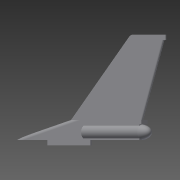
# Autodesk Inventor part: stabillizer
Saved by Autodesk Inventor 2014 SP1 (Build 180222100, 222)
## iProperties
Created: 2018-05-06
Part Number: stabillizer
Material: Generic
Document SubType Name: Modeling
Designer: Dadang
Density: 1 g/cm^3
Appearance: Default
Author: Dadang
Autodesk Inventor part; units mm, degrees
ref_plane "YZ Plane" through (0, 0, 0) normal (1, 0, 0) x (0, 1, 0)
ref_plane "XZ Plane" through (0, 0, 0) normal (0, 1, 0) x (-1, 0, 0)
sketch "Sketch1" plane through (0, 0, 0) normal (0, 0, 1) x (1, 0, 0)
  line L0 (0, 0) -> (330, 0)
  line L1 (0, 0) -> (0, 28)
  line L2 (0, 28) -> (-5, 28)
  line L3 (-5, 28) -> (-5, 36)
  line L4 (-5, 36) -> (183, 36)
  line L5 (183, 36) -> (330, 0)
  line L6 (-60, 191) -> (-60, 181)
  line L7 (-60, 181) -> (-55, 181)
  line L8 (-55, 181) -> (0, 36)
  line L9 (-60, 191) -> (25, 191)
  line L10 (33.5125, 187.4416) -> (183, 36)
  line L11 (25, 191) -> (33.5125, 187.4416)
  line L12 (242, 0) -> (242, -10)
  line L13 (242, -10) -> (132, -10)
  line L14 (132, -10) -> (132, 0)
  point P0 (30, 191)
  dimension "d0" = 330
  dimension "d1" = 28
  dimension "d2" = 5
  dimension "d3" = 8
  dimension "d4" = 188
  dimension "d7" = 10
  dimension "d8" = 5
  dimension "d9" = 90
  dimension "d10" = 88
  dimension "d11" = 10
  dimension "d12" = 110
  dimension "d23" = 145
  constraints: 30 end point, 5 point on line, 4 perpendicular, 3 parallel, 1 horizontal
  measures "d0" distance of L0.start L0.end
  measures "d1" distance of L0.start L1.end
  measures "d2" distance of L1.end L2.end
  measures "d3" distance of L2.end L3.end
  measures "d4" distance of L3.end L4.end
  measures "d7" distance of L6.start L6.end
  measures "d8" distance of L6.end L7.end
  measures "d9" distance of L6.start point (30, 191)
  measures "d10" distance of L0.end L12.start
  measures "d11" distance of L12.start L12.end
  measures "d12" distance of L12.end L13.end
  measures "d23" vertical distance of L7.end L8.end
extrude "Extrusion1" add sketch "Sketch1" along normal mid plane 16 contours L1 L2 L3 L4 L5 L0
extrude "Extrusion2" add sketch "Sketch1" along normal mid plane 5 contours L0 L12 L13 L14 | L4 L8 L7 L6 L9 L11 L10
fillet "Fillet1" radius 2.5 6 edges at (108.2563, 111.7208, 2.5) (108.2563, 111.7208, -2.5) (-60, 186, 2.5) (-60, 186, -2.5) (-27.5, 108.5, 2.5) (-27.5, 108.5, -2.5)
sketch "Sketch2" plane through (0, 0, 8) normal (0, -1, 0) x (1, 0, 0)
  line L0 (330, -16) -> (330, 0) projected
  line L1 (0, 0) -> (330, 0) projected
  line L2 (330, -16) -> (0, -16) projected
  line L3 (242, 0) -> (242, -16)
  line L4 (330, -8) -> (242, -8)
  line L5 (330, -8) -> (310.3863, -1.3058) construction
  line L6 (310.3863, -1.3058) -> (271.2053, 0) construction
  line L7 (271.2053, 0) -> (242, 0) construction
  spline S0 degree 3 poles (330, -8) (310.3863, -1.3058) (271.2053, 0) (242, 0) knots 1 1 1 1 2 2 2 2
  line L8 (330, -8) -> (310.3863, -14.6942) construction
  line L9 (310.3863, -14.6942) -> (271.2053, -16) construction
  line L10 (271.2053, -16) -> (242, -16) construction
  spline S1 degree 3 poles (330, -8) (310.3863, -14.6942) (271.2053, -16) (242, -16) knots 1 1 1 1 2 2 2 2
  line L11 (242, 0) -> (242, 7.2864)
  line L12 (242, 7.2864) -> (330, 7.2864)
  line L13 (330, 7.2864) -> (330, -26.6979)
  line L14 (330, -26.6979) -> (242, -26.6979)
  line L15 (242, -26.6979) -> (242, -16)
  point P0 (0, -8)
  constraints: 14 end point, 4 perpendicular, 4 point on line, 2 midpoint, 2 symmetric about line, 1 collinear, 1 parallel, 6 other
extrude "Extrusion3" cut sketch "Sketch2" against normal blind 50 contours L2 S1 L0 | L13 L14 L15 L2 | S0 L1 L0 | L1 L11 L12 L13
fillet "Fillet2" radius 7.9 4 edges at (212.5, 28.7755, 8) (286.2689, 10.7097, 6.7407) (212.5, 28.7755, -8) (286.2689, 10.7097, -6.7407)
sketch "Sketch3" plane through (0, 0, 8) normal (-1, 0, 0) x (0, 0, 1)
  circle A0 centre (-8, 14) radius 14
  point P0 (-8, 0)
  constraints: 1 vertical alignment, 2 other
extrude "Extrusion4" add sketch "Sketch3" along normal blind 20 and the other way blind 150
chamfer "Chamfer2" distance 5.9 angle 45 3 edges at (150, 14, -14) (150, 7.5193, 12.4097) (150, 20.4807, 12.4097)
ref_plane "Work Plane1" through (0, 0, 0) normal (0, 0, 1) x (1, 0, 0)
sketch "Sketch4" plane through (0, 0, 0) normal (0, 0, 1) x (1, 0, 0)
  line L0 (-20, 14) -> (-20, 20.9347) construction
  line L1 (-20, 20.9347) -> (-12.4443, 26.0318) construction
  line L2 (-12.4443, 26.0318) -> (0, 28) construction
  spline S0 degree 3 poles (-20, 14) (-20, 20.9347) (-12.4443, 26.0318) (0, 28) knots 1 1 1 1 2 2 2 2
  line L3 (-25.3833, 28) -> (-25.3833, 14)
  line L4 (-25.3833, 14) -> (-20, 14)
  line L5 (0, 28) -> (-25.3833, 28)
  line L6 (-20, 14) -> (-3.3131, 14)
  point P0 (0, 0)
  constraints: 8 end point, 2 parallel, 1 perpendicular, 3 other
revolve "Revolution1" cut sketch "Sketch4" angle 360 about axis through (-20, 14, 0) along (1, 0, 0)
body "Solid1"
